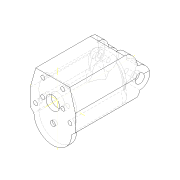
# Autodesk Inventor part: empty
Saved by Autodesk Inventor 2014 (Build 180170000, 170)
## iProperties
Created: 2015-04-13
Part Number: empty
Material: Generic
Document SubType Name: Modeling
Designer: Martin
Density: 1 g/cm^3
Appearance: Default
Author: Martin
Autodesk Inventor part; units mm, degrees
ref_plane "YZ Plane" through (0, 0, 0) normal (1, 0, 0) x (0, 1, 0)
ref_plane "XZ Plane" through (0, 0, 0) normal (0, 1, 0) x (-1, 0, 0)
ref_plane "XY Plane" through (0, 0, 0) normal (0, 0, 1) x (1, 0, 0)
sketch "sk_main" plane through (0, 0, 0) normal (1, 0, 0) x (0, 1, 0)
  line L0 (-10, 0) -> (42.5, 0) projected
  line L1 (0, -15.4) -> (0, 15.4) projected
  line L2 (25, -9) -> (0, -9)
  line L3 (0, -9) -> (0, 9)
  line L4 (0, 9) -> (25, 9)
  line L5 (25, 9) -> (25, -9)
  line L6 (25, -9) -> (0, 9) construction
  line L7 (0, -9) -> (25, 9) construction
  circle A0 centre (30, 0) radius 1
  circle A1 centre (30, 0) radius 5 construction
  line L8 (-2.5, 11) -> (30, 11)
  line L9 (30, 11) -> (30, 5)
  line L10 (30, -5) -> (30, -11)
  line L11 (30, -11) -> (-2.5, -11)
  line L12 (-2.5, -11) -> (-2.5, 11)
  arc A2 (30, -5) -> (30, 5) centre (30, 0) ccw
  line L13 (0, 11) -> (0, -11)
  line L14 (0, -11) -> (30, -11)
  line L15 (30, -11) -> (30, -9)
  line L16 (30, -9) -> (0, -9)
  line L17 (0, -9) -> (0, -11)
  line L18 (25, -5) -> (30, -5)
  line L19 (30, -5) -> (25, -5)
  line L20 (25, -5) -> (25, -9)
  line L21 (25, -9) -> (30, -9)
  line L22 (30, -9) -> (30, -5)
  point P0 (0, 0)
  point P1 (12.5, 0)
  dimension "d0" = 25
  dimension "d1" = 18
  dimension "d2" = 2
  dimension "d3" = 5
  dimension "d4" = 2
  dimension "d5" = 2.5
  dimension "d6" = 0
  constraints: 42 end point, 8 perpendicular, 8 point on line, 7 parallel, 4 point on circle, 3 centre point, 3 collinear, 3 horizontal, 2 midpoint, 2 tangent, 1 coincident, 1 concentric, 1 other
  measures "d0" distance of L3.end L4.end
  measures "d1" distance of L4.end L2.start
  measures "d2" diameter of A0
  measures "d3" distance from line of L5 A0.centre
  measures "d4" distance between parallel lines of L8 L4
  measures "d5" distance between parallel lines of L3 L12
  measures "d6" distance from line of A0.centre L9
extrude "ext_main_back" [suppressed]
extrude "ext_main_front" add sketch "sk_main" along normal mid plane 12.15 contours L12 L8 L1 L0 | L0 L1 L11 L12
sketch "sk_front" plane through (0, 0, 0) normal (0, 1, 0) x (-1, 0, 0)
  line L0 (0, -22.8535) -> (0, 18.1209) projected
  line L1 (15.9065, 0) -> (-15.9065, 0) projected
  circle A0 centre (0, 0) radius 3.4
  circle A1 centre (5.075, 0) radius 1
  circle A2 centre (-5.075, 0) radius 1
  circle A3 centre (0, 0) radius 8 construction
  circle A4 centre (0, -9) radius 8 construction
  circle A5 centre (0, -9) radius 1.25
  circle A6 centre (8.6494, -4.5) radius 1.75 construction
  circle A7 centre (-8.6494, -4.5) radius 1.75 construction
  line L2 (8.6494, -4.5) -> (-8.6494, -4.5) construction
  line L3 (-6.075, 11) -> (-6.075, -11) projected
  line L4 (6.075, -11) -> (6.075, 11) projected
  line L5 (10.3994, 1) -> (10.3994, -7) construction
  line L6 (10.3994, 1) -> (7.575, 11) construction
  line L7 (10.3994, -7) -> (6.075, -11) construction
  line L8 (-7.575, 11) -> (-10.3994, 1) construction
  line L9 (-10.3994, 1) -> (-10.3994, -7) construction
  line L10 (-10.3994, -7) -> (-6.075, -11) construction
  line L11 (6.075, -11) -> (-6.075, -11) projected
  circle A8 centre (-8.6494, -4.5) radius 1
  circle A9 centre (8.6494, -4.5) radius 1
  circle A10 centre (-5, 8.5) radius 1
  circle A11 centre (-5, 8.5) radius 2.25 construction
  line L12 (-5, 8.5) -> (5, 8.5) construction
  circle A12 centre (5, 8.5) radius 2.25 construction
  circle A13 centre (5, 8.5) radius 1
  line L13 (-6.075, 11) -> (-7.575, 11)
  line L14 (6.075, 11) -> (7.575, 11)
  line L15 (6.075, 11) -> (-6.075, 11) projected
  line L16 (-6.7285, -11.7065) -> (-11.3618, -7.4208)
  line L17 (-11.3618, -7.4208) -> (-11.3618, 1.1333)
  line L18 (-11.3618, 1.1333) -> (-8.2734, 12.068)
  line L19 (8.217, 12.2674) -> (11.3618, 1.1333)
  line L20 (11.3618, 1.1333) -> (11.3618, -7.4208)
  line L21 (11.3618, -7.4208) -> (6.7285, -11.7065)
  line L22 (-6.075, -11) -> (-7.4922, -11)
  line L23 (6.075, -11) -> (7.4922, -11)
  line L24 (-7.575, 11) -> (-8.575, 11)
  line L25 (7.575, 11) -> (8.575, 11)
  point P0 (0, 8.5)
  dimension "d11" = 6.8
  dimension "d12" = 2
  dimension "d13" = 10.15
  dimension "d14" = 16
  dimension "d15" = 16
  dimension "d16" = 9
  dimension "d17" = 2.5
  dimension "d18" = 3.5
  dimension "d21" = 8
  dimension "d22" = 4
  dimension "d26" = 2
  dimension "d27" = 2
  dimension "d28" = 4.5
  dimension "d30" = 10
  dimension "d31" = 8.5
  dimension "d37" = 1.5
  dimension "d42" = 1
  constraints: 40 end point, 14 centre point, 8 coincident, 8 point on line, 6 collinear, 5 tangent, 4 equal radius, 4 parallel, 4 perpendicular, 4 symmetric about line, 1 midpoint, 6 other
  measures "d11" diameter of A0
  measures "d12" diameter of A2
  measures "d13" distance of A2.centre A1.centre
  measures "d14" diameter of A3
  measures "d15" diameter of A4
  measures "d16" distance of A4.centre point (0, 0)
  measures "d17" diameter of A5
  measures "d18" diameter of A7
  measures "d21" distance of L5.start L5.end
  measures "d22" distance from line of L11 L5.end
  measures "d26" diameter of A9
  measures "d27" diameter of A10
  measures "d28" diameter of A11
  measures "d30" distance of L12.start L12.end
  measures "d31" distance between parallel lines of L1 L12
  measures "d37" distance of L3.start L8.start
  measures "d42" distance of L6.end L25.end
extrude "ext_front_tabs" add sketch "sk_front" against normal up to surface (2.5 mm away) contours L4 L1 L20 L21 L23 | L22 L16 L17 L1 L3 | L4 L14 L25 L19 L20 L1 | L1 L17 L18 L24 L13 L3 | A8 | A9
extrude "ext_cut_holesfront" cut sketch "sk_front" against normal through all contours A5 L0 | L0 A5 | A1 L1 | L1 A1 | A2 L1 | L1 A2 | A0 L1 L0 | L0 L1 A0 | L1 A0 L0 | L0 A0 L1 | A8 | A9 | A10 | A13
fillet "Fillet4" [suppressed]
extrude "ext_dowelfill" add sketch "sk_front" against normal blind 1.5 contours A5 L0 | L0 A5
extrude "Extrusion6" add sketch "sk_main" against normal up to surface (22.7235 mm away) from surface at 11.3618 contours L5 L4 L1 L8 L9 A2 L0 A0 | L0 A0 A2 L18 L5 | L18 L10 L16 L5
sketch "Sketch4" plane through (0, 0, 0) normal (0, 1, 0) x (-1, 0, 0)
  line L0 (9.1399, 9) -> (8.575, 11) projected
  line L1 (11.3618, 11) -> (8.575, 11) projected
  line L2 (11.3618, 11) -> (11.3618, 9) projected
  line L3 (11.3618, 9) -> (9.1399, 9) projected
  line L4 (-8.575, 11) -> (-9.1399, 9) projected
  line L5 (-9.1399, 9) -> (-11.3618, 9) projected
  line L6 (-11.3618, 9) -> (-11.3618, 11) projected
  line L7 (-8.575, 11) -> (-11.3618, 11) projected
  line L8 (11.3618, 9) -> (11.3618, -9) projected
  line L9 (-11.3618, -9) -> (11.3618, -9) projected
  line L10 (-11.3618, -9) -> (-11.3618, 9) projected
  line L11 (7.4922, -11) -> (11.3618, -7.4208) projected
  line L12 (-11.3618, -7.4208) -> (-7.4922, -11) projected
  line L13 (-9.1399, 9) -> (-11.3618, 1.1333) projected
  line L14 (11.3618, 1.1333) -> (9.1399, 9) projected
  line L15 (-11.3618, 11) -> (-8.575, 11)
  line L16 (-11.3618, 1.1333) -> (-8.575, 11)
  line L17 (-11.3618, 11) -> (-11.3618, 1.1333)
  line L18 (-11.3618, -7.4208) -> (-11.3618, -9)
  line L19 (-11.3618, -9) -> (-9.6544, -9)
  line L20 (-11.3618, -7.4208) -> (-9.6544, -9)
  line L21 (9.6544, -9) -> (11.3618, -7.4208)
  line L22 (11.3618, -7.4208) -> (11.3618, -9)
  line L23 (9.6544, -9) -> (11.3618, -9)
  line L24 (8.575, 11) -> (11.3618, 11)
  line L25 (11.3618, 1.1333) -> (11.3618, 11)
  line L26 (8.575, 11) -> (11.3618, 1.1333)
  constraints: 24 end point, 7 collinear, 4 perpendicular, 4 point on line
extrude "Extrusion7" cut sketch "Sketch4" along normal through all
sketch "Sketch5" plane through (0, 0, 0) normal (0, 1, 0) x (-1, 0, 0)
  circle A0 centre (-8.6494, -4.5) radius 1 projected
  circle A1 centre (0, 0) radius 3.4 projected
  circle A2 centre (-5.075, 0) radius 1 projected
  circle A3 centre (5.075, 0) radius 1 projected
  circle A4 centre (8.6494, -4.5) radius 1 projected
  line L0 (9.1399, 9) -> (5.866, 9) projected
  arc A5 (4.134, 9) -> (5.866, 9) centre (5, 8.5) ccw projected
  line L1 (4.134, 9) -> (-4.134, 9) projected
  arc A6 (-5.866, 9) -> (-4.134, 9) centre (-5, 8.5) ccw projected
  line L2 (-5.866, 9) -> (-9.1399, 9) projected
  line L3 (-9.1399, 9) -> (-11.3618, 1.1333) projected
  line L4 (-11.3618, 1.1333) -> (-11.3618, -7.4208) projected
  line L5 (-11.3618, -7.4208) -> (-7.4922, -11) projected
  line L6 (7.4922, -11) -> (-7.4922, -11) projected
  line L7 (7.4922, -11) -> (11.3618, -7.4208) projected
  line L8 (11.3618, -7.4208) -> (11.3618, 1.1333) projected
  line L9 (11.3618, 1.1333) -> (9.1399, 9) projected
  line L10 (0, -15.2468) -> (0, 14.4809) projected
  circle A7 centre (0, 0) radius 9.5
  line L11 (3.0414, 9) -> (9.1399, 9)
  line L12 (9.1399, 9) -> (11.3618, 1.1333)
  line L13 (11.3618, 1.1333) -> (11.3618, -7.4208)
  line L14 (-9.6544, -9) -> (9.6544, -9) projected
  circle A8 centre (0, 0) radius 9 construction
  line L15 (9, 0) -> (9, -9) construction
  line L16 (9, -3.0414) -> (9, -9)
  line L17 (9, -9) -> (9.6544, -9)
  line L18 (11.3618, -7.4208) -> (9.6544, -9)
  arc A9 (9, -3.0414) -> (3.0414, 9) centre (0, 0) ccw
  line L19 (-9, 0) -> (-9, -9.6054) construction
  line L20 (-9, -3.0414) -> (-9, -9)
  line L21 (-9, -9) -> (-9.6544, -9)
  line L22 (-3.0414, 9) -> (-9.1399, 9)
  line L23 (-11.3618, 1.1333) -> (-9.1399, 9)
  line L24 (-11.3618, 1.1333) -> (-11.3618, -7.4208)
  line L25 (-11.3618, -7.4208) -> (-9.6544, -9)
  arc A10 (-3.0414, 9) -> (-9, -3.0414) centre (0, 0) ccw
  dimension "d43" = 19
  dimension "d44" = 18
  constraints: 28 end point, 10 point on circle, 9 point on line, 7 collinear, 5 perpendicular, 4 centre point, 3 concentric, 2 coincident, 2 tangent
  measures "d43" diameter of A7
  measures "d44" diameter of A8
extrude "Extrusion8" add sketch "Sketch5" along normal up to surface (25 mm away) contours L20 A0 | A0 L20 L14 L5 L4 L3 L2 A6 A7 | A6 L22 A7 | A6 L1 A7 | L16 A4 A7 A5 L0 L9 L8 L7 L14 | L16 A4 | L1 A5 A7 | L11 A5 A7
sketch "Sketch6" plane through (-10.2697, 30, 5) normal (0, 1, 0) x (1, 0, 0)
  line L0 (1.6947, -6) -> (18.8447, -6) projected
  line L1 (2.7774, 16) -> (17.7619, 16) projected
  line L2 (10.2697, 16) -> (10.2697, -6) construction
  line L3 (14.7697, -6) -> (14.7697, 16)
  line L4 (14.7697, 16) -> (5.7697, 16)
  line L5 (5.7697, 16) -> (5.7697, -6)
  line L6 (5.7697, -6) -> (14.7697, -6)
  line L7 (14.7697, -6) -> (5.7697, 16) construction
  line L8 (14.7697, 16) -> (5.7697, -6) construction
  point P0 (10.2697, 5)
  point P1 (10.2697, 5)
  dimension "d47" = 9
  constraints: 14 end point, 5 midpoint, 3 parallel, 2 point on line, 1 perpendicular
  measures "d47" distance between parallel lines of L5 L3
extrude "Extrusion9" cut sketch "Sketch6" along normal blind 5 and the other way blind 5
sketch "Sketch7" plane through (0, 0, 0) normal (0, 1, 0) x (-1, 0, 0)
  line L0 (7.4922, -11) -> (-7.4922, -11) projected
  circle A0 centre (0, -9) radius 1.25 projected
  line L1 (-9.6544, -9) -> (-7.4922, -11) projected
  line L2 (7.4922, -11) -> (9.6544, -9) projected
  circle A1 centre (0, -9) radius 8.5 construction
  circle A2 centre (0, -9) radius 9.5
  line L3 (-9.4989, -9.1439) -> (-7.4922, -11)
  line L4 (9.4989, -9.1439) -> (7.4922, -11)
  line L5 (7.4922, -11) -> (-7.4922, -11)
  point P0 (0, 0)
  dimension "d52" = 17
  dimension "d53" = 1
  constraints: 6 end point, 2 centre point, 2 coincident, 2 collinear, 2 point on circle, 2 point on line
  measures "d52" diameter of A1
  measures "d53" radial gap between concentric circles of A2 A1
extrude "ext_gear2_bottomcover" add sketch "Sketch7" against normal up to surface (2.5 mm away) contours L2 A2 L1 L0 picked at (-0.378, -13.4774)
fillet "Fillet5" radius 5 4 edges at (-6.5375, 30, 11) (6.5375, 30, 11) (7.0772, 30, -9) (-7.0772, 30, -9)
sketch "Sketch8" plane through (11.3618, -2.5, 1.1333) normal (1, 0, 0) x (0, 0, -1)
  circle A0 centre (1.1333, 32.5) radius 1 projected
  arc A1 (6.1333, 32.5) -> (0, 37.3699) centre (1.1333, 32.5) ccw projected
  circle A2 centre (1.1333, 32.5) radius 2.25
  point P0 (1.1333, 2.5)
  dimension "d57" = 4.5
  constraints: 1 centre point, 1 coincident
  measures "d57" diameter of A2
extrude "ext_cut_screwhead" cut sketch "Sketch8" against normal blind 2.5 contours A0 | A2
mirror "Mirror1" about plane through (0, 0, 0) normal (1, 0, 0) of "ext_cut_screwhead"
sketch "Sketch10" plane through (0, 0, 0) normal (1, 0, 0) x (0, 1, 0)
  circle A0 centre (30, 0) radius 1 projected
  arc A1 (25.101, -9) -> (30, -5) centre (25.101, -4) ccw projected
  arc A2 (30, -5) -> (30, 5) centre (30, 0) ccw projected
  line L0 (30, 6) -> (30, 5) projected
  arc A3 (30, 6) -> (25, 11) centre (25, 6) ccw projected
  line L1 (25, 11) -> (25, 8.3666) projected
  line L2 (25, -9) -> (25, 8.3666) projected
  line L3 (25.101, -9) -> (25, -9) projected
  line L4 (25, 6) -> (25, -9)
  arc A4 (25, -9) -> (28.5, -7.667) centre (25.0987, -3.9977) ccw
  arc A5 (28.5, -7.667) -> (25, 6) centre (-3.4871, -8.5769) ccw
  point P0 (0, 0)
  dimension "d65" = 15
  dimension "d66" = 3.5
  dimension "d67" = 32
  constraints: 5 point on circle, 2 centre point, 2 end point, 1 collinear, 1 point on line
  measures "d65" distance of L4.start L2.start
  measures "d66" horizontal distance of A4.end L2.start
  measures "d67" radius of A5
extrude "ext_cut_motorcutway" cut sketch "Sketch10" along normal up to surface (18 mm away) from surface at -9 contours L3 L2 A5 A1
fillet "Fillet7" radius 5 2 edges at (9, 27.5126, -0.6382) (-9, 27.5126, -0.6382)
equation "\"d2\" = screw_m2_bore_selfthreading"
equation "\"d12\" = screw_m2_bore_selfthreading"
equation "\"d26\" = screw_m2_bore_selfthreading"
equation "\"d27\" = screw_m2_bore_selfthreading"
equation "\"d28\" = screw_m2_head_maxsize"
equation "\"d48\" = d3"
equation "\"d49\" = d3"
equation "\"d54\" = d3"
equation "\"d57\" = screw_m2_head_maxsize"
equation "\"screw_m2_bore_selfthreading\" = 2"
equation "\"screw_m2_head_maxsize\" = 4.5"
body "Solid1"
